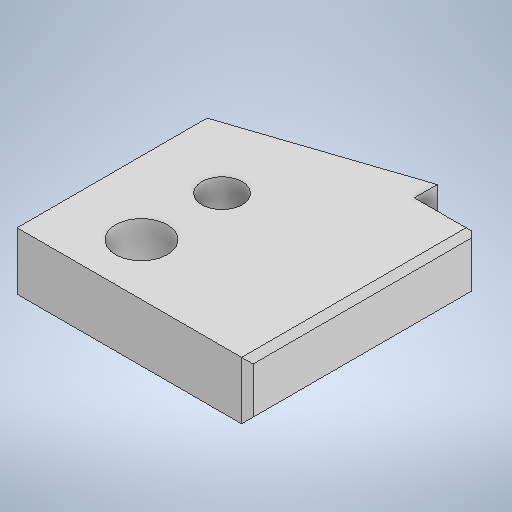
# Autodesk Inventor part: 21-30-220-B3
Saved by Autodesk Inventor 2025.2 (Build 292293000, 293)
## iProperties
Created: 2024-11-14
Part Number: 21-30-220-B3
Material: Generic
Document SubType Name: Modeling
Designer: Zvonko.Gabric
Density: 1 g/cm^3
Appearance: Default
Author: Zvonko.Gabric
Autodesk Inventor part; units mm, degrees
ref_plane "YZ Plane" through (0, 0, 0) normal (1, 0, 0) x (0, 1, 0)
ref_plane "XZ Plane" through (0, 0, 0) normal (0, 1, 0) x (-1, 0, 0)
ref_plane "XY Plane" through (0, 0, 0) normal (0, 0, 1) x (1, 0, 0)
sketch "Sketch1" plane through (0, 0, 0) normal (0, 1, 0) x (-1, 0, 0)
  line L0 (0, 0) -> (0, -16.5)
  line L1 (0, -16.5) -> (-15, -21.5)
  line L2 (-15, -21.5) -> (-15, -20)
  line L3 (-15, -20) -> (-20, -20)
  line L4 (-20, -20) -> (-20, 0)
  line L5 (-20, 0) -> (0, 0)
  circle A0 centre (-6.3, -4.5) radius 2.25
  circle A1 centre (-6.3, -11.5) radius 1.75
  point P0 (-15, -20.75)
  dimension "d0" = 16.5
  dimension "d1" = 20
  dimension "d2" = 20
  dimension "d3" = 21.5
  dimension "d4" = 5
  dimension "d5" = 4.5
  dimension "d6" = 11.5
  dimension "d7" = 4.5
  dimension "d8" = 3.5
  dimension "d9" = 13.7
  dimension "d10" = 13.7
  constraints: 12 end point, 3 perpendicular, 2 centre point, 1 midpoint, 1 parallel, 1 vertical
  measures "d0" distance of L0.start L0.end
  measures "d1" distance between parallel lines of L4 L0
  measures "d2" distance of L3.end L4.end
  measures "d3" distance from line of L5 L1.end
  measures "d4" distance from line of point (-15, -20.75) L4
  measures "d5" distance from line of L5 A0.centre
  measures "d6" distance from line of L5 A1.centre
  measures "d7" diameter of A0
  measures "d8" diameter of A1
  measures "d9" distance from line of L4 A0.centre
  measures "d10" distance from line of L4 A1.centre
extrude "Extrusion1" add sketch "Sketch1" along normal blind 5
chamfer "Chamfer1" distance 0.5 angle 45 2 edges at (17.5, 0, -20) (20, 0, -10) measured on face at (15.9997, 0, -10.3604)
chamfer "Chamfer2" distance 0.5 angle 45 2 edges at (17.5, 5, -20) (20, 5, -10) measured on face at (15.9997, 5, -10.3604)
chamfer "Chamfer3" distance 0.5 angle 45 2 edges at (20, 2.5, -20) (20, 2.5, 0) measured on face at (20, 3.1667, -13.3333)
body "Solid1"
